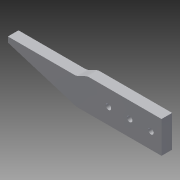
# Autodesk Inventor part: Y_shaft_support_brace
Saved by Autodesk Inventor 2013 (Build 170138000, 138)
## iProperties
Created: 2013-09-23
Part Number: Y_shaft_support_brace
Material: Aluminum 6061
Document SubType Name: Modeling
Designer: Ian
Density: 2.71 g/cm^3
Mass: 182.257 g
Surface Area: 166.697 cm^2
Volume: 67.2535 cm^3
d8: 0.500 in
d9: 0.00 deg
d25: 0.500 in
d26: 0.750 in
d27: 3.235 in
d30: 8.000 in
d32: 6.000 in
d34: 4.000 in
d35: 1.500 in
d36: 1.500 in
d37: 1.000 in
d38: 1.000 in
d39: 0.500 in
d98: 0.250 in
d100: 0.500 in
d101: 63.43 deg
d102: 72.82 deg
d103: 1.500 in
d104: 0.250 in
d105: 3.117 in
d106: 0.257 in
Author: Ian
Autodesk Inventor part; units mm, degrees
ref_plane "YZ Plane" through (0, 0, 0) normal (1, 0, 0) x (0, 1, 0)
ref_plane "XZ Plane" through (0, 0, 0) normal (0, 1, 0) x (-1, 0, 0)
ref_plane "XY Plane" through (0, 0, 0) normal (0, 0, 1) x (1, 0, 0)
sketch "Sketch1" plane through (0, 0, 0) normal (0, 0, 1) x (1, 0, 0)
  line L0 (0, 0) -> (0, -12.7) construction
  line L1 (0, -12.7) -> (0, -31.75) construction
  line L2 (0, 6.35) -> (0, 0) construction
  line L3 (-50.8, -19.05) -> (152.4, -19.05) construction
  line L4 (82.169, 0) -> (183.769, 0) construction
  line L5 (183.769, 0) -> (183.769, -38.1) construction
  line L6 (183.769, -38.1) -> (82.169, -38.1) construction
  line L7 (82.169, -38.1) -> (82.169, 0) construction
  line L8 (183.769, 0) -> (183.769, -38.1)
  line L9 (183.769, -38.1) -> (82.169, -38.1)
  line L10 (79.1709, -6.35) -> (0, -6.35) construction
  line L11 (0, -6.35) -> (0, -12.7)
  line L12 (0, -12.7) -> (82.169, -38.1)
  line L13 (0, -6.35) -> (79.1709, -6.35)
  line L14 (97.8671, 0) -> (183.769, 0)
  line L15 (84.8505, -5.0092) -> (92.1875, -1.3408)
  arc A0 (79.1709, -6.35) -> (84.8505, -5.0092) centre (79.1709, 6.35) ccw
  arc A1 (97.8671, 0) -> (92.1875, -1.3408) centre (97.8671, -12.7) ccw
  point P0 (120.269, -19.05)
  point P1 (145.669, -19.05)
  point P2 (171.069, -19.05)
  dimension "d25" = 12.7
  dimension "d26" = 19.05
  dimension "d27" = 82.169
  dimension "d30" = 203.2
  dimension "d32" = 152.4
  dimension "d34" = 101.6
  dimension "d35" = 38.1
  dimension "d36" = 38.1
  dimension "d37" = 25.4
  dimension "d38" = 25.4
  dimension "d39" = 12.7
  dimension "d98" = 6.35
  dimension "d100" = 12.7
  dimension "d101" = 63.435
  dimension "d102" = 72.823
  dimension "d103" = 38.1
  dimension "d104" = 6.35
  dimension "d105" = 79.1709
  constraints: 32 end point, 5 perpendicular, 5 point on line, 4 collinear, 4 point on circle, 4 tangent, 3 parallel, 2 centre point, 1 equal radius, 1 horizontal, 1 midpoint, 1 vertical
  measures "d25" distance of L0.start L0.end
  measures "d26" distance of L0.end L1.end
  measures "d27" distance of L0.start L4.start
  measures "d30" distance of L3.start L3.end
  measures "d32" distance from line of L3.end L0
  measures "d34" distance of L5.end L6.end
  measures "d35" distance of L4.end L5.end
  measures "d36" distance from line of L7 point (120.269, -19.05)
  measures "d37" distance of point (120.269, -19.05) point (145.669, -19.05)
  measures "d38" distance of point (145.669, -19.05) point (171.069, -19.05)
  measures "d39" distance from line of L8 point (171.069, -19.05)
  measures "d98" distance from line of L0.start L10
  measures "d100" radius of A0
  measures "d101" angle of L15 L5
  measures "d102" angle of L12 L5
  measures "d103" diameter of L14 L3
  measures "d104" distance from line of L2.start L14
  measures "d105" distance from line of L0 A0.centre
extrude "Extrusion1" add sketch "Sketch1" against normal blind 12.7
hole "Hole7" at (120.269, -19.05, 0) at (145.669, -19.05, 0) at (171.069, -19.05, 0) direction (0, 0, -1) diameter 6.5278 end through all clearance for "Socket Head Cap Screw" size "1/4" standard "Ansi Unified Screw Threads"
body "Solid1"
